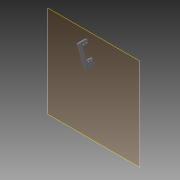
# Autodesk Inventor part: servoMountPlate
Saved by Autodesk Inventor 2013 (Build 170138000, 138)
## iProperties
Created: 2014-08-20
Part Number: servoMountPlate
Material: Generic
Document SubType Name: Modeling
Designer: Nano
Density: 1 g/cm^3
Author: Nano
Autodesk Inventor part; units mm, degrees
ref_plane "YZ Plane" through (0, 0, 0) normal (1, 0, 0) x (0, 1, 0)
ref_plane "XZ Plane" through (0, 0, 0) normal (0, 1, 0) x (-1, 0, 0)
ref_plane "XY Plane" through (0, 0, 0) normal (0, 0, 1) x (1, 0, 0)
ref_plane "Work Plane1" through (0, 0, 0) normal (0, 0, 1) x (1, 0, 0)
sketch "Sketch1" plane through (0, 0, 0) normal (0, 0, 1) x (1, 0, 0)
  line L0 (0, 152.4) -> (-45.5982, 133.5126) projected
  line L1 (-31.4153, 139.3873) -> (-25.5487, 141.8174)
  line L2 (-25.5487, 141.8174) -> (3.6118, 71.4178)
  line L3 (3.6118, 71.4178) -> (-2.2548, 68.9877)
  line L4 (-2.2548, 68.9877) -> (-31.4153, 139.3873)
  point P0 (0, 0)
  dimension "d0" = 6.35
  dimension "d1" = 76.2
  constraints: 8 end point, 2 parallel, 1 perpendicular
  measures "d0" distance of L1.start L1.end
  measures "d1" distance of L1.end L2.end
extrude "Extrusion1" add sketch "Sketch1" along normal blind 31.75
sketch "Sketch2" plane through (-25.5487, 141.8174, 31.75) normal (0.9238795, 0.3826834, 0) x (0, 0, -1)
  line L0 (11.43, -52.324) -> (11.43, -13.716) projected
  line L1 (30.734, -53.34) -> (12.446, -53.34) projected
  line L2 (12.446, -12.7) -> (20.955, -12.7) projected
  line L3 (11.43, -53.34) -> (11.43, -12.7)
  line L4 (11.43, -12.7) -> (31.75, -12.7)
  line L5 (31.75, -12.7) -> (31.75, -53.34)
  line L6 (31.75, -53.34) -> (11.43, -53.34)
  point P0 (31.75, -140.7992)
  constraints: 8 end point, 2 parallel, 1 perpendicular
extrude "Extrusion2" cut sketch "Sketch2" against normal through all
sketch "Sketch3" plane through (-25.5487, 141.8174, 31.75) normal (0.9238795, 0.3826834, 0) x (0, 0, -1)
  arc A0 (18.161, -58.6942) -> (14.859, -58.6942) centre (16.51, -57.15) ccw projected
  arc A1 (28.321, -58.6942) -> (25.019, -58.6942) centre (26.67, -57.15) ccw projected
  arc A2 (14.859, -7.3458) -> (18.161, -7.3458) centre (16.51, -8.89) ccw projected
  arc A3 (25.019, -7.3458) -> (28.321, -7.3458) centre (26.67, -8.89) ccw projected
  circle A4 centre (16.51, -57.15) radius 2.2606
  circle A5 centre (26.67, -57.15) radius 2.2606
  circle A6 centre (16.51, -8.89) radius 2.2606
  circle A7 centre (26.67, -8.89) radius 2.2606
  point P0 (31.75, -140.7992)
  constraints: 4 centre point
extrude "Extrusion3" cut sketch "Sketch3" against normal through all
sketch "Sketch4" plane through (0, 0, 0) normal (0, 0, -1) x (-1, 0, 0)
  line L0 (11.003, 90.1076) -> (5.1363, 92.5377) construction
  line L1 (5.1363, 92.5377) -> (-3.6118, 71.4178) construction
  line L2 (-3.6118, 71.4178) -> (2.2548, 68.9877) construction
  line L3 (2.2548, 68.9877) -> (11.003, 90.1076) construction
  line L4 (20.6886, 130.0841) -> (26.5552, 127.6541) construction
  line L5 (26.5552, 127.6541) -> (31.4153, 139.3873) construction
  line L6 (31.4153, 139.3873) -> (25.5487, 141.8174) construction
  line L7 (25.5487, 141.8174) -> (20.6886, 130.0841) construction
  line L8 (24.224, 138.6194) -> (21.794, 132.7528)
  line L9 (21.794, 132.7528) -> (27.6606, 130.3227)
  line L10 (27.6606, 130.3227) -> (30.0907, 136.1894)
  line L11 (30.0907, 136.1894) -> (24.224, 138.6194)
  line L12 (4.1298, 90.1076) -> (1.6998, 84.241)
  line L13 (1.6998, 84.241) -> (7.5664, 81.8109)
  line L14 (7.5664, 81.8109) -> (9.9964, 87.6776)
  line L15 (9.9964, 87.6776) -> (4.1298, 90.1076)
  line L16 (-0.2443, 79.5477) -> (-2.6743, 73.681)
  line L17 (-2.6743, 73.681) -> (3.1923, 71.251)
  line L18 (3.1923, 71.251) -> (5.6224, 77.1176)
  line L19 (5.6224, 77.1176) -> (-0.2443, 79.5477)
  point P0 (0, 0)
  dimension "d8" = 6.35
  dimension "d9" = 6.35
  dimension "d10" = 6.35
  dimension "d11" = 6.35
  dimension "d12" = 6.35
  constraints: 24 end point, 6 parallel, 3 perpendicular
  measures "d8" distance of L8.start L8.end
  measures "d9" distance of L9.end L8.end
  measures "d10" distance of L12.start L12.end
  measures "d11" distance of L13.end L12.end
  measures "d12" distance of L16.start L16.end
extrude "Extrusion4" add sketch "Sketch4" along normal blind 3.175
body "Solid1"
